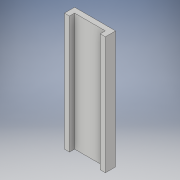
# Autodesk Inventor part: rev1 tube
Saved by Autodesk Inventor 2017 (Build 210142000, 142)
## iProperties
Created: 2019-05-04
Part Number: rev1 tube
Material: Generic
Document SubType Name: Modeling
Designer: Roman
Density: 1 g/cm^3
Appearance: Default
Author: Roman
Autodesk Inventor part; units mm, degrees
ref_plane "YZ Plane" through (0, 0, 0) normal (1, 0, 0) x (0, 1, 0)
ref_plane "XZ Plane" through (0, 0, 0) normal (0, 1, 0) x (-1, 0, 0)
ref_plane "XY Plane" through (0, 0, 0) normal (0, 0, 1) x (1, 0, 0)
sketch "Sketch1" plane through (0, 0, 0) normal (0, 0, 1) x (1, 0, 0)
  line L0 (0, 0) -> (203.2, 0)
  line L1 (203.2, 0) -> (203.2, -584.2)
  line L2 (203.2, -584.2) -> (0, -584.2)
  line L3 (0, -584.2) -> (0, 0)
  dimension "d0" = 203.2
  dimension "d1" = 584.2
  constraints: 8 end point, 2 parallel, 1 horizontal, 1 perpendicular
  measures "d0" distance of L1.end L2.end
  measures "d1" distance of L0.end L1.end
extrude "Extrusion1" add sketch "Sketch1" along normal blind 25.4
sketch "Sketch2" plane through (0, 0, 25.4) normal (0, 0, 1) x (1, 0, 0)
  line L0 (0, -584.2) -> (203.2, -584.2) projected
  line L1 (0, 0) -> (25.4, 0)
  line L2 (25.4, 0) -> (25.4, -584.2)
  line L3 (25.4, -584.2) -> (0, -584.2)
  line L4 (0, -584.2) -> (0, 0)
  line L5 (203.2, 0) -> (0, 0) projected
  line L6 (203.2, 0) -> (177.8, 0)
  line L7 (177.8, 0) -> (177.8, -584.2)
  line L8 (177.8, -584.2) -> (203.2, -584.2)
  line L9 (203.2, -584.2) -> (203.2, 0)
  dimension "d4" = 25.4
  dimension "d5" = 25.4
  dimension "d6" = 584.2
  constraints: 16 end point, 4 parallel, 2 horizontal, 2 perpendicular, 1 point on line
  measures "d4" distance of L2.end L3.end
  measures "d5" distance of L8.end L7.end
  measures "d6" distance of L7.end L6.end
extrude "Extrusion2" add sketch "Sketch2" along normal blind 25.4 contours L4 L1 L2 L0 | L7 L5 L9 L0
body "Solid1"
